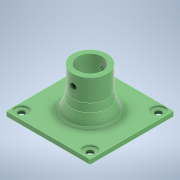
# Autodesk Inventor part: Soporte_Vertical_Para_Balancin
Saved by Autodesk Inventor 2022 (Build 260153000, 153)
## iProperties
Created: 2022-01-24
Part Number: Soporte_Vertical_Para_Balancin
Material: ABS Plastic
Document SubType Name: Modeling
Designer: hurta
Density: 1.06 g/cm^3
Appearance: Smooth - Dark Forest Green
Author: hurta
Autodesk Inventor part; units mm, degrees
ref_plane "YZ Plane" through (0, 0, 0) normal (1, 0, 0) x (0, 1, 0)
ref_plane "XZ Plane" through (0, 0, 0) normal (0, 1, 0) x (-1, 0, 0)
ref_plane "XY Plane" through (0, 0, 0) normal (0, 0, 1) x (1, 0, 0)
sketch "Sketch1" plane through (0, 0, 0) normal (0, 1, 0) x (-1, 0, 0)
  circle A0 centre (0, 0) radius 22.5
  line L0 (55, -55) -> (-55, -55)
  line L1 (-55, -55) -> (-55, 55)
  line L2 (-55, 55) -> (55, 55)
  line L3 (55, 55) -> (55, -55)
  line L4 (55, -55) -> (-55, 55) construction
  line L5 (-55, -55) -> (55, 55) construction
  circle A1 centre (0, 0) radius 16.4
  dimension "d0" = 45
  dimension "d1" = 110
  dimension "d2" = 110
  dimension "d3" = 32.8
  constraints: 12 end point, 2 centre point, 2 coincident, 2 midpoint, 2 parallel, 1 horizontal, 1 perpendicular
  measures "d0" diameter of A0
  measures "d1" distance of L1.end L2.end
  measures "d2" distance of L0.end L1.end
  measures "d3" diameter of A1
extrude "Extrusion1" add sketch "Sketch1" along normal blind 6 contours L0 L1 L2 L3
extrude "Extrusion2" add sketch "Sketch1" along normal blind 60 contours A0
chamfer "Chamfer1" distance 10 angle 45 1 edges at (22.5, 6, 0)
sketch "Sketch3" plane through (0, 6, 0) normal (0, 1, 0) x (1, 0, 0)
  line L0 (55, -55) -> (55, 55) projected
  line L1 (55, 55) -> (-55, 55) projected
  line L2 (-55, -55) -> (55, -55) projected
  line L3 (-55, 55) -> (-55, -55) projected
  point P0 (0, 0)
  point P1 (-45, 45)
  point P2 (-45, -45)
  point P3 (45, -45)
  point P4 (45, 45)
  point P5 (55, 0)
  point P6 (0, 55)
  point P7 (0, -55)
  point P8 (-55, 0)
  dimension "d14" = 10
  dimension "d15" = 10
  dimension "d16" = 10
  dimension "d17" = 10
  constraints: 2 horizontal alignment, 2 vertical alignment
  measures "d14" distance from line of point (45, 45) L0
  measures "d15" distance from line of point (45, 45) L1
  measures "d16" distance from line of L2 point (-45, -45)
  measures "d17" distance from line of L3 point (-45, -45)
hole "Hole1" at (-45, 6, -45) at (45, 6, -45) at (45, 6, 45) at (-45, 6, 45) direction (0, -1, 0) diameter 8.5 end through all counterbore diameter 18.01 counterbore depth 2 clearance for "Hex Head Bolt" size "M8" standard "Ansi Metric M Profile"
sketch "Sketch4" plane through (-55, 0, 55) normal (0, 0, 1) x (1, 0, 0)
  line L0 (0, 0) -> (110, 0) projected
  line L1 (77.5, 60) -> (32.5, 60) projected
  point P0 (55, 0)
  point P1 (55, 45)
  point P2 (55, 0)
  dimension "d25" = 15
  constraints: 1 midpoint, 1 vertical alignment
  measures "d25" distance from line of L1 point (55, 45)
hole "Hole2" at (0, 45, 55) direction (0, 0, -1) diameter 8.5 end through all clearance for "Hex Head Bolt" size "M8" standard "Ansi Metric M Profile"
chamfer "Chamfer2" distance 10 angle 45 1 edges at (22.5, 16, 0)
chamfer "Chamfer3" distance 5 angle 45 1 edges at (22.5, 26, 0)
body "Solid1"
